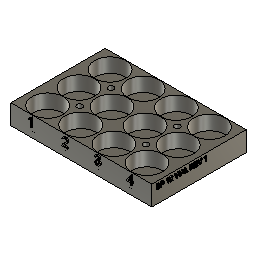
20cc_vial_plate v5 (Autodesk Fusion 360 design; units mm, degrees)
Autodesk Fusion 360 part; units mm, degrees
sketch "Sketch1" plane through (0, 0, 0) normal (0, 0, 1) x (1, 0, 0)
  line L0 (0, 0) -> (127.76, 0)
  line L1 (127.76, 0) -> (127.76, -85.48)
  line L2 (127.76, -85.48) -> (0, -85.48)
  line L3 (0, -85.48) -> (0, 0)
  dimension "d1" = 127.76
  dimension "d2" = 85.48
  constraint horizontal L0
  constraint vertical L1
  constraint horizontal L2
  constraint vertical L3
  constraint coincident L0.start L3.end
  measures "d1" distance of L0.start L0.end
  measures "d2" distance of L0.start L2.end
extrude "Extrude1" add sketch "Sketch1" along normal blind 18
sketch "Sketch7" plane through (0, 0, 18) normal (0, 0, 1) x (-1, 0, 0)
  line L0 (0, 85.48) -> (-127.76, 85.48)
  line L1 (-127.76, 85.48) -> (-127.76, 0)
  line L2 (-127.76, 0) -> (0, 0)
  line L3 (0, 0) -> (0, 85.48)
  point P0 (-18.875, 14.4325)
  point P1 (-48.878, 14.4325)
  point P2 (-78.881, 14.4325)
  point P3 (-108.884, 14.4325)
  point P4 (-18.875, 42.74)
  point P5 (-48.878, 42.74)
  point P6 (-78.881, 42.74)
  point P7 (-108.884, 42.74)
  point P8 (-18.875, 71.0475)
  point P9 (-48.878, 71.0475)
  point P10 (-78.881, 71.0475)
  point P11 (-108.884, 71.0475)
  dimension "d42" = -30.003
  dimension "d43" = 28.3075
hole "Hole1" at (18.875, -14.4325, 18) at (18.875, -42.74, 18) at (18.875, -71.0475, 18) at (48.878, -71.0475, 18) at (48.878, -42.74, 18) at (48.878, -14.4325, 18) at (78.881, -14.4325, 18) at (78.881, -42.74, 18) at (78.881, -71.0475, 18) at (108.884, -71.0475, 18) at (108.884, -42.74, 18) at (108.884, -14.4325, 18) direction (0, 0, -1) diameter 28.1 depth 13 tip angle 180
sketch "Sketch3" plane through (0, -85.48, 0) normal (0, -1, 0) x (1, 0, 0)
  line L0 (0, 0) -> (127.76, 0)
  line L1 (127.76, 0) -> (127.76, 18)
  line L2 (127.76, 18) -> (0, 18)
  line L3 (0, 18) -> (0, 0)
  line L4 (14.0494, 7.6995) -> (23.0494, 7.6995) construction
  line L5 (23.0494, 7.6995) -> (23.0494, 16.6995) construction
  line L6 (23.0494, 16.6995) -> (14.0494, 16.6995) construction
  line L7 (14.0494, 16.6995) -> (14.0494, 7.6995) construction
  line L8 (46.9022, 9.8546) -> (52.4077, 9.8546) construction
  line L9 (52.4077, 9.8546) -> (52.4077, 16.3088) construction
  line L10 (52.4077, 16.3088) -> (46.9022, 16.3088) construction
  line L11 (46.9022, 16.3088) -> (46.9022, 9.8546) construction
  line L12 (76.5166, 10.3535) -> (82.0221, 10.3535) construction
  line L13 (82.0221, 10.3535) -> (82.0221, 16.8078) construction
  line L14 (82.0221, 16.8078) -> (76.5166, 16.8078) construction
  line L15 (76.5166, 16.8078) -> (76.5166, 10.3535) construction
  line L16 (106.4547, 1.2473) -> (111.5714, 1.3263) construction
  line L17 (111.5714, 1.3263) -> (111.3033, 18.6919) construction
  line L18 (111.3033, 18.6919) -> (106.1865, 18.6129) construction
  line L19 (106.1865, 18.6129) -> (106.4547, 1.2473) construction
  dimension "d12" = 8
  dimension "d13" = 8
  dimension "d14" = 8
  dimension "d15" = 8
  text T0 "1" font "Arial" height 8 align centre top in box 9 x 9 at (14.0494, 7.6995) x (1, 0) y (0, 1) spacing 1 kerned
  text T1 "2" font "Arial" height 8 align centre top in box 5.5055 x 6.4543 at (46.9022, 9.8546) x (1, 0) y (0, 1) spacing 1 kerned
  text T2 "3" font "Arial" height 8 align centre top in box 5.5055 x 6.4543 at (76.5166, 10.3535) x (1, 0) y (0, 1) spacing 1 kerned
  text T3 "4" font "Arial" height 8 align centre top in box 5.1174 x 17.3677 at (106.4547, 1.2473) x (0.999881, 0.01544) y (-0.01544, 0.999881) spacing 1 kerned
extrude "Extrude2" add sketch "Sketch3" along normal blind 1 text T0 T1 T2 T3
sketch "Sketch4" plane through (0, 0, 0) normal (-1, 0, 0) x (0, -1, 0)
  line L0 (0, 0) -> (85.48, 0)
  line L1 (85.48, 0) -> (85.48, 18)
  line L2 (85.48, 18) -> (0, 18)
  line L3 (0, 18) -> (0, 0)
  line L4 (9.6912, 7.6466) -> (15.9169, 7.6466) construction
  line L5 (15.9169, 7.6466) -> (15.9169, 16.9806) construction
  line L6 (15.9169, 16.9806) -> (9.6912, 16.9806) construction
  line L7 (9.6912, 16.9806) -> (9.6912, 7.6466) construction
  line L8 (40.0437, 6.0325) -> (46.2694, 6.0325) construction
  line L9 (46.2694, 6.0325) -> (46.2694, 15.3665) construction
  line L10 (46.2694, 15.3665) -> (40.0437, 15.3665) construction
  line L11 (40.0437, 15.3665) -> (40.0437, 6.0325) construction
  line L12 (70.6777, 8.7329) -> (70.6779, 8.7329) construction
  line L13 (70.6779, 8.7329) -> (70.9216, 18.0676) construction
  line L14 (70.9216, 18.0676) -> (70.9213, 18.0676) construction
  line L15 (70.9213, 18.0676) -> (70.6777, 8.7329) construction
  dimension "d23" = 8
  dimension "d24" = 8
  dimension "d26" = 8
  text T0 "A" font "Arial" height 8 align centre top in box 6.2257 x 9.334 at (9.6912, 7.6466) x (1, 0) y (0, 1) spacing 1 kerned
  text T1 "B" font "Arial" height 8 align centre top in box 6.2257 x 9.334 at (40.0437, 6.0325) x (1, 0) y (0, 1) spacing 1 kerned
extrude "Extrude3" add sketch "Sketch4" along normal blind 1 text T0 T1
sketch "Sketch5" plane through (127.76, 0, 0) normal (1, 0, 0) x (0, 1, 0)
  line L0 (-85.48, 0) -> (0, 0)
  line L1 (0, 0) -> (0, 18)
  line L2 (0, 18) -> (-85.48, 18)
  line L3 (-85.48, 18) -> (-85.48, 0)
  line L4 (-82.6452, 7.4287) -> (-35.8624, 7.5304) construction
  line L5 (-35.8624, 7.5304) -> (-35.8813, 16.2534) construction
  line L6 (-35.8813, 16.2534) -> (-82.6642, 16.1518) construction
  line L7 (-82.6642, 16.1518) -> (-82.6452, 7.4287) construction
  dimension "d32" = 4
  text T0 "BP 12 VIAL REV 1" font "Arial" height 4 align centre top in box 46.783 x 8.7231 at (-82.6452, 7.4287) x (0.999998, 0.002173) y (-0.002173, 0.999998) spacing 1 kerned
extrude "Extrude4" add sketch "Sketch5" along normal blind 1 text T0
sketch "Sketch6" plane through (0, 0, 18) normal (0, 0, 1) x (-1, 0, 0)
  line L0 (0, 85.48) -> (-127.76, 85.48)
  line L1 (-127.76, 85.48) -> (-127.76, 0)
  line L2 (-127.76, 0) -> (0, 0)
  line L3 (0, 0) -> (0, 85.48)
  circle A0 centre (-108.884, 42.74) radius 14.05
  circle A1 centre (-78.881, 71.0475) radius 14.05
  circle A2 centre (-78.881, 14.4325) radius 14.05
  circle A3 centre (-48.878, 42.74) radius 14.05
  circle A4 centre (-18.875, 71.0475) radius 14.05
  circle A5 centre (-18.875, 14.4325) radius 14.05
  circle A6 centre (-18.875, 42.74) radius 14.05
  circle A7 centre (-48.878, 71.0475) radius 14.05
  circle A8 centre (-48.878, 14.4325) radius 14.05
  circle A9 centre (-78.881, 42.74) radius 14.05
  circle A10 centre (-108.884, 71.0475) radius 14.05
  circle A11 centre (-108.884, 14.4325) radius 14.05
  point P0 (-33.8765, 28.587)
  point P1 (-93.8825, 28.587)
  point P2 (-33.8765, 56.8945)
  point P3 (-93.8825, 56.8945)
  dimension "d46" = -60.006
  dimension "d47" = 28.3075
hole "Hole2" at (33.8765, -28.587, 18) at (33.8765, -56.8945, 18) at (93.8825, -28.587, 18) at (93.8825, -56.8945, 18) direction (0, 0, -1) diameter 3.4 depth 20 tip angle 180 counterbore diameter 5.1 counterbore depth 8
fillet "Fillet1" [no effect]
